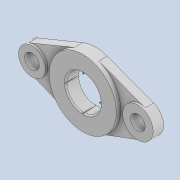
# Autodesk Inventor part: 0.5in Flanged Pillowblock Frame
Saved by Autodesk Inventor 2022 (Build 260153000, 153)
## iProperties
Created: 2021-10-10
Part Number: 0.5in Flanged Pillowblock Frame
Material: Generic
Document SubType Name: Modeling
Designer: Coy
Density: 1 g/cm^3
Appearance: Default
Author: Coy
Autodesk Inventor part; units mm, degrees
ref_plane "YZ Plane" through (0, 0, 0) normal (1, 0, 0) x (0, 1, 0)
ref_plane "XZ Plane" through (0, 0, 0) normal (0, 1, 0) x (-1, 0, 0)
ref_plane "XY Plane" through (0, 0, 0) normal (0, 0, 1) x (1, 0, 0)
sketch "Sketch1" plane through (0, 0, 0) normal (0, 0, 1) x (1, 0, 0)
  circle A0 centre (0, 0) radius 6.35
  line L0 (0, 0) -> (-20, 0) construction
  line L1 (0, 0) -> (20, 0) construction
  circle A1 centre (-20, 0) radius 2.75
  circle A2 centre (20, 0) radius 2.75
  arc A3 (-21.9405, 4.7385) -> (-21.9405, -4.7385) centre (-20, 0) ccw
  arc A4 (21.9978, -5.3861) -> (21.9978, 5.3861) centre (20, 0) ccw
  line L2 (-21.9405, 4.7385) -> (-4.813, 11.7527)
  line L3 (-21.9405, -4.7385) -> (-4.813, -11.7527)
  line L4 (4.4166, -11.9073) -> (21.9978, -5.3861)
  line L5 (4.4166, 11.9073) -> (21.9978, 5.3861)
  arc A5 (4.4166, 11.9073) -> (-4.813, 11.7527) centre (0, 0) ccw
  arc A6 (-4.813, -11.7527) -> (4.4166, -11.9073) centre (0, 0) ccw
  dimension "d0" = 12.7
  dimension "d2" = 20
  dimension "d3" = 20
  dimension "d4" = 5.5
  dimension "d5" = 5.5
  constraints: 12 end point, 8 point on circle, 8 tangent, 7 centre point, 6 coincident, 2 horizontal
  measures "d0" diameter of A0
  measures "d2" distance of L0.start L0.end
  measures "d3" distance of L0.start L1.end
  measures "d4" diameter of A1
  measures "d5" diameter of A2
extrude "Extrusion1" add sketch "Sketch1" along normal blind 4.7625
chamfer "Chamfer1" distance 4.7625 angle 2 1 edges at (-6.35, 0, 4.7625) measured on face at (-6.35, 0, 4.2625)
sketch "Sketch2" plane through (0, 0, 4.7625) normal (0, 0, 1) x (1, 0, 0)
  line L0 (0.2, 6.5132) -> (0.2, 6.3468)
  line L1 (-0.2, 6.5132) -> (-0.2, 6.3468)
  circle A0 centre (0, 0) radius 6.5163 projected
  circle A1 centre (0, 0) radius 6.35 projected
  arc A2 (-0.2, 6.3532) -> (0.2, 6.3532) centre (0, 6.35) ccw
  line L2 (-6.5132, -0.2) -> (-6.3468, -0.2)
  arc A3 (-6.3532, -0.2) -> (-6.3532, 0.2) centre (-6.35, 0) ccw
  line L3 (-6.5132, 0.2) -> (-6.3468, 0.2)
  line L4 (0.2, -6.5132) -> (0.2, -6.3468)
  arc A4 (0.2, -6.3532) -> (-0.2, -6.3532) centre (0, -6.35) ccw
  line L5 (-0.2, -6.5132) -> (-0.2, -6.3468)
  line L6 (6.5132, 0.2) -> (6.3468, 0.2)
  arc A5 (6.3532, 0.2) -> (6.3532, -0.2) centre (6.35, 0) ccw
  line L7 (6.5132, -0.2) -> (6.3468, -0.2)
  dimension "d11" = 0.2
  dimension "d12" = 0.2
  dimension "d15" = 360
  constraints: 16 end point, 16 point on circle, 8 point on line, 4 centre point, 2 vertical, 41 other
  measures "d11" distance from line of point (0, 0) L0
  measures "d12" distance from line of point (0, 0) L1
extrude "Extrusion2" add sketch "Sketch2" against normal blind 4.7625 contours L0 A1 L1 A0 | A0 L7 A5 A1 L6 | A2 A1 | L3 A3 A1 L2 A0 | A1 A5 | A3 A1 | A0 L5 A4 A1 L4 | A1 A4
fillet "Fillet1" radius 0.5 4 edges at (-4.6077, 4.6077, 4.7625) (-4.6077, -4.6077, 4.7625) (4.6077, -4.6077, 4.7625) (4.6077, 4.6077, 4.7625)
sketch "Sketch3" plane through (0, 0, 4.7625) normal (0, 0, 1) x (1, 0, 0)
  circle A0 centre (0, 0) radius 12.7
  circle A1 centre (20, 0) radius 2.75 projected
  circle A2 centre (-20, 0) radius 2.75 projected
  line L0 (-4.813, 11.7527) -> (-21.9405, 4.7385) projected
  arc A3 (-21.9405, 4.7385) -> (-21.9405, -4.7385) centre (-20, 0) ccw projected
  line L1 (-21.9405, -4.7385) -> (-4.813, -11.7527) projected
  arc A4 (-4.813, -11.7527) -> (4.4166, -11.9073) centre (0, 0) ccw projected
  line L2 (4.4166, -11.9073) -> (21.9978, -5.3861) projected
  arc A5 (21.9978, -5.3861) -> (21.9978, 5.3861) centre (20, 0) ccw projected
  line L3 (21.9978, 5.3861) -> (4.4166, 11.9073) projected
  arc A6 (4.4166, 11.9073) -> (-4.813, 11.7527) centre (0, 0) ccw projected
  line L4 (0.2, 6.3468) -> (0.2, 6.9963) projected
  arc A7 (6.9963, 0.2) -> (0.2, 6.9963) centre (0, 0) ccw projected
  line L5 (6.9963, 0.2) -> (6.3468, 0.2) projected
  arc A8 (6.3468, 0.2) -> (6.3468, -0.2) centre (6.35, 0) ccw projected
  line L6 (6.3468, -0.2) -> (6.9963, -0.2) projected
  arc A9 (0.2, -6.9963) -> (6.9963, -0.2) centre (0, 0) ccw projected
  line L7 (0.2, -6.9963) -> (0.2, -6.3468) projected
  arc A10 (0.2, -6.3468) -> (-0.2, -6.3468) centre (0, -6.35) ccw projected
  line L8 (-0.2, -6.3468) -> (-0.2, -6.9963) projected
  arc A11 (-6.9963, -0.2) -> (-0.2, -6.9963) centre (0, 0) ccw projected
  line L9 (-6.9963, -0.2) -> (-6.3468, -0.2) projected
  arc A12 (-6.3468, -0.2) -> (-6.3468, 0.2) centre (-6.35, 0) ccw projected
  line L10 (-6.3468, 0.2) -> (-6.9963, 0.2) projected
  arc A13 (-0.2, 6.9963) -> (-6.9963, 0.2) centre (0, 0) ccw projected
  line L11 (-0.2, 6.9963) -> (-0.2, 6.3468) projected
  arc A14 (-0.2, 6.3468) -> (0.2, 6.3468) centre (0, 6.35) ccw projected
  point P0 (4.4166, -11.9073)
  constraints: 1 centre point, 1 coincident
extrude "Extrusion3" cut sketch "Sketch3" against normal blind 1.5875 contours A0 L3 A5 L2 | A0 L1 A3 L0
sketch "Sketch4" plane through (0, 0, 3.175) normal (0, 0, 1) x (1, 0, 0)
  circle A0 centre (-20, 0) radius 2.75 projected
  circle A1 centre (20, 0) radius 2.75 projected
  circle A2 centre (-20, 0) radius 5.1205
  circle A3 centre (20, 0) radius 5.7447
  point P0 (0, 0)
  constraints: 2 centre point, 2 coincident
extrude "Extrusion4" add sketch "Sketch4" along normal blind 0.7937
equation "\"d5\" = d4"
body "Solid1"
